Autodesk Inventor part; units mm, degrees
(part 2 of 2)
  spline S73 degree 2 poles (3.0646, -124.0746) (3.7616, -123.3084) (4.2708, -122.3889) (4.2708, -121.8996) knots 0 0 0 1 2 2 2
  spline S74 degree 2 poles (4.2708, -121.8996) (4.2708, -121.6425) (4.1126, -121.2569) (3.9692, -121.1334) knots 0 0 0 1 2 2 2
  spline S75 degree 2 poles (3.9692, -121.1334) (3.8259, -121.0098) (3.4502, -120.8862) (3.2228, -120.8862) knots 0 0 0 1 2 2 2
  spline S76 degree 2 poles (3.2228, -120.8862) (3.0053, -120.8862) (2.5604, -120.9949) (2.3577, -121.079) knots 0 0 0 1 2 2 2
  spline S77 degree 2 poles (2.3577, -121.079) (2.1847, -121.1482) (1.8634, -121.3459) (1.7645, -121.4151) knots 0 0 0 1 2 2 2
  line L413 (1.7645, -121.4151) -> (1.72, -121.4151)
  line L414 (1.72, -121.4151) -> (1.72, -120.5451)
  spline S78 degree 2 poles (1.72, -120.5451) (1.9721, -120.4215) (2.8768, -120.1793) (3.2821, -120.1793) knots 0 0 0 1 2 2 2
  spline S79 degree 2 poles (3.2821, -120.1793) (4.1373, -120.1793) (5.1012, -121.0839) (5.1012, -121.8551) knots 0 0 0 1 2 2 2
  spline S80 degree 2 poles (5.1012, -121.8551) (5.1012, -122.2159) (4.9332, -122.819) (4.7849, -123.0761) knots 0 0 0 1 2 2 2
  spline S81 degree 2 poles (4.7849, -123.0761) (4.6366, -123.343) (4.2065, -123.867) (3.9692, -124.1191) knots 0 0 0 1 2 2 2
  spline S82 degree 2 poles (3.9692, -124.1191) (3.5836, -124.5393) (2.6395, -125.4389) (2.3577, -125.7009) knots 0 0 0 1 2 2 2
  line L415 (2.3577, -125.7009) -> (5.3533, -125.7009)
  line L416 (5.3533, -125.7009) -> (5.3533, -126.4078)
  line L417 (20.189, -126.4078) -> (16.6546, -126.4078)
  line L418 (16.6546, -126.4078) -> (16.6546, -120.3078)
  line L419 (16.6546, -120.3078) -> (17.4653, -120.3078)
  line L420 (17.4653, -120.3078) -> (17.4653, -125.6861)
  line L421 (17.4653, -125.6861) -> (20.189, -125.6861)
  line L422 (20.189, -125.6861) -> (20.189, -126.4078)
  spline S83 degree 2 poles (22.2998, -120.8862) (22.0773, -120.8862) (21.6374, -120.9949) (21.4248, -121.079) knots 0 0 0 1 2 2 2
  spline S84 degree 2 poles (21.4248, -121.079) (21.2271, -121.163) (20.9354, -121.341) (20.8217, -121.4201) knots 0 0 0 1 2 2 2
  line L423 (20.8217, -121.4201) -> (20.7723, -121.4201)
  line L424 (20.7723, -121.4201) -> (20.7723, -120.555)
  spline S85 degree 2 poles (20.7723, -120.555) (21.0392, -120.4116) (21.9538, -120.1793) (22.364, -120.1793) knots 0 0 0 1 2 2 2
  spline S86 degree 2 poles (22.364, -120.1793) (22.7793, -120.1793) (23.3972, -120.3474) (23.6493, -120.5253) knots 0 0 0 1 2 2 2
  spline S87 degree 2 poles (23.6493, -120.5253) (23.9162, -120.7181) (24.1931, -121.2767) (24.1931, -121.6524) knots 0 0 0 1 2 2 2
  spline S88 degree 2 poles (24.1931, -121.6524) (24.1931, -122.1566) (23.5307, -122.9179) (23.066, -123.0167) knots 0 0 0 1 2 2 2
  line L425 (23.066, -123.0167) -> (23.066, -123.0761)
  spline S89 degree 2 poles (23.066, -123.0761) (23.2588, -123.1156) (23.6987, -123.2936) (23.8866, -123.4715) knots 0 0 0 1 2 2 2
  spline S90 degree 2 poles (23.8866, -123.4715) (24.0744, -123.6445) (24.3117, -124.1982) (24.3117, -124.5986) knots 0 0 0 1 2 2 2
  spline S91 degree 2 poles (24.3117, -124.5986) (24.3117, -125.0089) (24.0299, -125.7059) (23.7729, -125.9728) knots 0 0 0 1 2 2 2
  spline S92 degree 2 poles (23.7729, -125.9728) (23.5059, -126.2496) (22.7496, -126.5364) (22.2701, -126.5364) knots 0 0 0 1 2 2 2
  spline S93 degree 2 poles (22.2701, -126.5364) (21.8104, -126.5364) (20.9107, -126.3139) (20.6042, -126.1607) knots 0 0 0 1 2 2 2
  line L426 (20.6042, -126.1607) -> (20.6042, -125.2956)
  line L427 (20.6042, -125.2956) -> (20.6636, -125.2956)
  spline S94 degree 2 poles (20.6636, -125.2956) (20.9206, -125.4834) (21.7906, -125.8295) (22.2207, -125.8295) knots 0 0 0 1 2 2 2
  spline S95 degree 2 poles (22.2207, -125.8295) (22.4728, -125.8295) (22.977, -125.6713) (23.1451, -125.4884) knots 0 0 0 1 2 2 2
  spline S96 degree 2 poles (23.1451, -125.4884) (23.3082, -125.3055) (23.4812, -124.8705) (23.4812, -124.5393) knots 0 0 0 1 2 2 2
  spline S97 degree 2 poles (23.4812, -124.5393) (23.4812, -124.2081) (23.2884, -123.778) (23.1154, -123.6544) knots 0 0 0 1 2 2 2
  spline S98 degree 2 poles (23.1154, -123.6544) (22.9424, -123.5308) (22.4728, -123.4369) (22.196, -123.4369) knots 0 0 0 1 2 2 2
  line L428 (22.196, -123.4369) -> (21.8499, -123.4369)
  line L429 (21.8499, -123.4369) -> (21.8499, -122.7597)
  line L430 (21.8499, -122.7597) -> (22.1218, -122.7597)
  spline S99 degree 2 poles (22.1218, -122.7597) (22.6705, -122.7597) (23.3626, -122.2357) (23.3626, -121.7364) knots 0 0 0 1 2 2 2
  spline S100 degree 2 poles (23.3626, -121.7364) (23.3626, -121.5041) (23.1846, -121.1729) (23.0413, -121.074) knots 0 0 0 1 2 2 2
  spline S101 degree 2 poles (23.0413, -121.074) (22.888, -120.9702) (22.5123, -120.8862) (22.2998, -120.8862) knots 0 0 0 1 2 2 2
  point P0 (0, 0)
  dimension "d68" = 4
  dimension "d69" = 15
  dimension "d70" = 145
  dimension "d73" = 25
  dimension "d83" = 25
  dimension "d148" = 19.5
  dimension "d150" = 1
  dimension "d157" = 19.5
  dimension "d176" = 50
  dimension "d177" = 62
  dimension "d178" = 20
  dimension "d179" = 1
  dimension "d180" = 1
  dimension "d181" = 1
  dimension "d182" = 1
  dimension "d183" = 1
  dimension "d184" = 1
  constraints: 240 end point, 18 parallel, 9 horizontal, 9 perpendicular, 4 horizontal alignment, 1 point on line, 195 other
  measures "d68" distance between parallel lines of L3 L1
  measures "d69" distance between parallel lines of L0 L2
  measures "d70" distance between parallel lines of L5 L1
  measures "d73" distance of L1.start L6.start
  measures "d83" distance of L38.start L42.end
  measures "d148" distance between parallel lines of L63 L65
  measures "d150" distance between parallel lines of L63 L66
  measures "d157" distance of L62.end L71.end
  measures "d176" distance between parallel lines of L123 L125
  measures "d177" distance between parallel lines of L127 L123
  measures "d178" distance between parallel lines of L131 L133
  measures "d179" distance between parallel lines of L122 L134
  measures "d180" distance between parallel lines of L126 L142
  measures "d181" distance between parallel lines of L123 L145
  measures "d182" distance between parallel lines of L127 L143
  measures "d183" distance between parallel lines of L128 L144
  measures "d184" distance between parallel lines of L130 L138
extrude "Extrusion4" cut sketch "Sketch5" against normal blind 1 contours L1 L2 L3 L0 | L6 L8 L7 L9 | L10 L12 L11 L13 | L14 L16 L15 L17 | L18 L20 L19 L21 | L22 L24 L23 L25 | L26 L28 L27 L29 | L30 L32 L31 L33 | L34 L36 L35 L37 | L38 L40 L39 L41 | L42 L45 L44 L43 | L46 L49 L48 L47 | L50 L53 L52 L51 | L54 L57 L56 L55 | L62 L63 L64 L65 | L71 L74 L76 L63 | L79 L82 L84 L74 | L87 L90 L92 L82 | L95 L98 L100 L90 | L158 A1 L159 A0 L160 A2 | L164 L165 L166 L167 L168 L169 L170 L171 L172 L173 L174 | L175 L176 L177 L178 L179 L180 L181 L182 L183 L184 L185 L186 L187 | L188 L189 L190 L191 L192 L193 L194 L195 | L199 L200 L201 L202 L203 L204 L205 S0 S1 S2 L206 | L210 L211 L212 L213 L214 L215 L216 L217 L218 L219 | L220 L221 L222 L223 L224 L225 L226 L227 L228 L229 L230 L231 | L232 L233 L234 L235 L236 L237 L238 L239 L240 L241 | S7 S8 S9 S10 S11 S12 L242 L243 S13 S14 S15 S16 S17 S18 L244 L245 L246 L247 L248 S19 S20 | L249 L250 L251 L252 | L253 L254 L255 L256 | L257 L258 L259 L260 L261 L262 L263 L264 L265 L266 L267 L268 | L269 L270 L271 L272 L273 L274 L275 L276 L277 L278 L279 L280 | S21 S22 S23 S24 S25 S26 L281 L282 S27 S28 S29 S30 S31 S32 L283 L284 L285 L286 L287 S33 S34 | L288 L289 L290 L291 L292 L293 L294 L295 L296 L297 L298 L299 | L300 L301 L302 L303 L304 L305 L306 | S35 S36 S37 S38 S39 S40 S41 S42 | L307 L308 L309 L310 L311 L312 | L313 L314 L315 L316 L317 L318 L319 L320 | L321 L322 L323 L324 L325 L326 L327 L328 | S49 S50 S51 S52 S53 S54 L332 L333 S55 S56 S57 S58 S59 S60 L334 L335 L336 L337 L338 S61 S62 | L339 L340 L341 L342 L343 L344 L345 L346 L347 L348 L349 L350 | L351 L352 L353 L354 | L355 L356 L357 L358 | S63 S64 L359 L360 L361 L362 L363 S65 S66 | L367 L368 L369 L370 L371 L372 L373 L374 L375 L376 L377 L378 | L379 L380 L381 L382 L383 L384 L385 L386 L387 L388 | L389 L390 L391 L392 L393 L394 | L395 L396 L397 L398 L399 L400 S71 L401 L402 L403 L404 | L405 L406 L407 L408 L409 L410 | L411 L412 S72 S73 S74 S75 S76 S77 L413 L414 S78 S79 S80 S81 S82 L415 L416 | L417 L418 L419 L420 L421 L422 | S83 S84 L423 L424 S85 S86 S87 S88 L425 S89 S90 S91 S92 S93 L426 L427 S94 S95 S96 S97 S98 L428 L429 L430 S99 S100 S101
equation "\"d2\" = 0.5 * d1"
equation "\"d3\" = 0.5 * d0"
body "Solid1"
